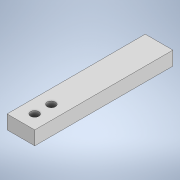
# Autodesk Inventor part: Soporte3_Dos
Saved by Autodesk Inventor 2021 (Build 250183000, 183)
## iProperties
Created: 2023-12-04
Part Number: Soporte3_Dos
Material: Generic
Document SubType Name: Modeling
Designer: Nicol
Density: 1 g/cm^3
Appearance: Default
Author: Nicol
Autodesk Inventor part; units mm, degrees
ref_plane "YZ Plane" through (0, 0, 0) normal (1, 0, 0) x (0, 1, 0)
ref_plane "XZ Plane" through (0, 0, 0) normal (0, 1, 0) x (-1, 0, 0)
ref_plane "XY Plane" through (0, 0, 0) normal (0, 0, 1) x (1, 0, 0)
sketch "Sketch1" plane through (0, 0, 0) normal (0, 1, 0) x (-1, 0, 0)
  line L0 (0, 0) -> (10, 0)
  line L1 (10, 0) -> (10, -50)
  line L2 (10, -50) -> (0, -50)
  line L3 (0, -50) -> (0, 0)
  circle A0 centre (5, -5) radius 1.5
  circle A1 centre (5, -11) radius 1.5
  dimension "d0" = 10
  dimension "d1" = 50
  dimension "d4" = 3
  dimension "d5" = 3
  dimension "d6" = 6
  dimension "d7" = 5
  dimension "d8" = 5
  constraints: 8 end point, 2 centre point, 2 parallel, 1 horizontal, 1 perpendicular
  measures "d0" distance of L1.end L2.end
  measures "d1" distance of L0.end L1.end
  measures "d4" diameter of A0
  measures "d5" diameter of A1
  measures "d6" distance of A1.centre A0.centre
  measures "d7" distance from line of L0 A0.centre
  measures "d8" distance from line of L3 A0.centre
extrude "Extrusion2" add sketch "Sketch1" along normal blind 5
body "Solid2"
